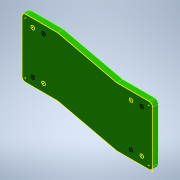
# Autodesk Inventor part: DB2_Bridge
Saved by Autodesk Inventor 2021 (Build 250183000, 183)
## iProperties
Created: 2020-04-05
Part Number: DB2_Bridge
Material: Generic
Document SubType Name: Modeling
Designer: lgnds
Density: 1 g/cm^3
Appearance: Default
Author: lgnds
Autodesk Inventor part; units mm, degrees
ref_plane "YZ Plane" through (0, 0, 0) normal (1, 0, 0) x (0, 1, 0)
ref_plane "XZ Plane" through (0, 0, 0) normal (0, 1, 0) x (-1, 0, 0)
ref_plane "XY Plane" through (0, 0, 0) normal (0, 0, 1) x (1, 0, 0)
sketch "Sketch1" plane through (0, 0, 0) normal (0, 0, 1) x (1, 0, 0)
  line L0 (0, 0) -> (0, 16.5)
  line L1 (0, 16.5) -> (-10, 16.5)
  line L2 (-10, 16.5) -> (-26.5, 20.348)
  line L3 (-26.5, 20.348) -> (-36.5, 20.348)
  line L4 (-36.5, 20.348) -> (-36.5, 3.848)
  line L5 (-36.5, 3.848) -> (-26.5, 3.848)
  line L6 (-26.5, 3.848) -> (-10, 0)
  line L7 (-10, 0) -> (0, 0)
  dimension "d0" = 10
  dimension "d1" = 10
  dimension "d2" = 10
  dimension "d3" = 10
  dimension "d4" = 3.848
  dimension "d5" = 36.5
  dimension "d6" = 16.5
  constraints: 16 end point, 3 parallel, 3 perpendicular, 1 vertical
  measures "d0" distance of L0.end L1.end
  measures "d1" distance of L2.end L3.end
  measures "d2" distance of L4.end L5.end
  measures "d3" distance of L6.end L0.start
  measures "d4" distance between parallel lines of L1 L3
  measures "d5" distance between parallel lines of L0 L4
  measures "d6" distance between parallel lines of L5 L3
extrude "Extrusion1" add sketch "Sketch1" along normal blind 1.6
sketch "Sketch2" plane through (0, 0, 1.6) normal (0, 0, 1) x (1, 0, 0)
  line L0 (-7.4638, 8.25) -> (0, 8.25)
  line L1 (0, 0) -> (0, 16.5) projected
  line L2 (-36.5, 20.348) -> (-36.5, 3.848) projected
  line L3 (-36.5, 12.098) -> (-30.2249, 12.098)
  line L4 (-26.5, 20.348) -> (-36.5, 20.348) projected
  line L5 (-31.9735, 20.348) -> (-31.9735, 3.848)
  line L6 (-4.5265, 16.5) -> (-4.5265, 0)
  line L7 (-10, 0) -> (0, 0) projected
  line L8 (0, 16.5) -> (-10, 16.5) projected
  dimension "d9" = 16.5
  dimension "d12" = 27.447
  dimension "d13" = 36.5
  dimension "d14" = 4.5265
  constraints: 8 end point, 2 horizontal, 2 midpoint, 2 point on line, 1 perpendicular, 1 vertical
  measures "d9" distance between parallel lines of L8 L7
  measures "d12" distance between parallel lines of L5 L6
  measures "d13" distance between parallel lines of L1 L2
  measures "d14" distance between parallel lines of L5 L2
fillet "Fillet1" radius 1 4 edges at (-36.5, 20.348, 0.8) (-36.5, 3.848, 0.8) (0, 0, 0.8) (0, 16.5, 0.8)
sketch "OUTLINE" plane through (0, 0, 1.6) normal (0, 0, 1) x (1, 0, 0)
  arc A0 (0, 15.5) -> (-1, 16.5) centre (-1, 15.5) ccw projected
  line L0 (-1, 16.5) -> (-10, 16.5) projected
  line L1 (-10, 16.5) -> (-26.5, 20.348) projected
  line L2 (-26.5, 20.348) -> (-35.5, 20.348) projected
  arc A1 (-35.5, 20.348) -> (-36.5, 19.348) centre (-35.5, 19.348) ccw projected
  line L3 (-36.5, 19.348) -> (-36.5, 4.848) projected
  arc A2 (-36.5, 4.848) -> (-35.5, 3.848) centre (-35.5, 4.848) ccw projected
  line L4 (-35.5, 3.848) -> (-26.5, 3.848) projected
  line L5 (-26.5, 3.848) -> (-10, 0) projected
  line L6 (-10, 0) -> (-1, 0) projected
  arc A3 (-1, 0) -> (0, 1) centre (-1, 1) ccw projected
  line L7 (0, 1) -> (0, 15.5) projected
  point P0 (0, 0)
sketch "EXTRA" plane through (0, 0, 1.6) normal (0, 0, 1) x (1, 0, 0)
  circle A0 centre (-3.0265, 2.25) radius 0.49 projected
  circle A1 centre (-6.0265, 14.25) radius 0.49 projected
  circle A2 centre (-30.4735, 6.098) radius 0.5193 projected
  circle A3 centre (-33.4735, 18.098) radius 0.5193 projected
  circle A4 centre (-6.0265, 2.25) radius 0.49
  circle A5 centre (-3.0265, 14.25) radius 0.49
  circle A6 centre (-30.4735, 18.098) radius 0.49
  circle A7 centre (-33.4735, 6.098) radius 0.49
  point P0 (0, 0)
  constraints: 4 centre point, 8 other
equation "\"d1\" = d0"
equation "\"d2\" = d1"
equation "\"d3\" = d0"
equation "\"d14\" = -0.5 * d12 + 0.5 * d13"
body "Solid1"
